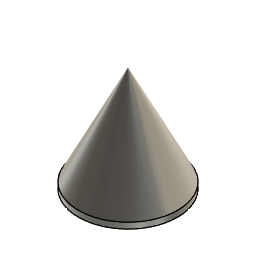
Topic-2-Fusion (Autodesk Fusion 360 design; units mm, degrees)
Autodesk Fusion 360 part; units mm, degrees
sketch "Sketch1" plane through (0, 0, 0) normal (0, 0, 1) x (1, 0, 0)
  circle A0 centre (0, 0) radius 25
  dimension "d1" = 50
  constraint coincident A0.centre origin
  measures "d1" diameter of A0
ref_plane "WorkPlane1" through (0, 0, 50) normal (0, 0, 1) x (1, 0, 0)
sketch "Sketch2" plane through (0, 0, 50) normal (0, 0, 1) x (1, 0, 0)
loft "Loft1" add profiles "Sketch1" section 1 section 2 point at (0, 0, 50)
shell "Shell1" thickness 3 removed faces 1 at (2.6796, -11.7401, 0)
sketch "Sketch3" plane through (0, 0, 0) normal (0, 0, 1) x (1, 0, 0)
  circle A0 centre (0, 0) radius 10
  circle A1 centre (0, 0) radius 25
  circle A2 centre (0, 0) radius 21.6459
  dimension "d4" = 20
  constraint coincident A0.centre A1.centre
  measures "d4" diameter of A0
extrude "Extrude1" add sketch "Sketch3" against normal blind 3 contours A1 | A2
